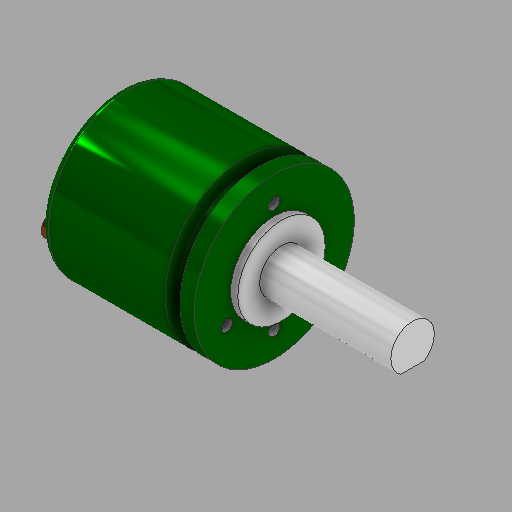
# Autodesk Inventor part: Энкодер P3022-V1-CW360
Saved by Autodesk Inventor 2025 (Build 290162000, 162)
## iProperties
Created: 2025-04-07
Part Number: Энкодер P3022-V1-CW360
Material: Типовые
Document SubType Name: Modeling
Designer: Artem Sannikov
Density: 1 g/cm^3
Appearance: По умолчанию
Author: Artem Sannikov
Autodesk Inventor part; units mm, degrees
ref_plane "YZ Plane" through (0, 0, 0) normal (1, 0, 0) x (0, 1, 0)
ref_plane "XZ Plane" through (0, 0, 0) normal (0, 1, 0) x (-1, 0, 0)
ref_plane "XY Plane" through (0, 0, 0) normal (0, 0, 1) x (1, 0, 0)
sketch "Эскиз1" plane through (0, 0, 0) normal (0, 0, 1) x (1, 0, 0)
  line L0 (0, 0) -> (19.3512, 0) construction
  line L1 (0, 0) -> (0, 11)
  line L2 (0, 11) -> (17, 11)
  line L3 (17, 11) -> (17, 9)
  line L4 (17, 11) -> (17, 9)
  line L5 (17, 9) -> (19, 9)
  line L6 (19, 9) -> (19, 11)
  line L7 (19, 11) -> (21, 11)
  line L8 (21, 11) -> (21, 6)
  line L9 (0, 0) -> (16.5209, 0)
  line L10 (21, 6) -> (22, 6)
  line L11 (22, 6) -> (22, 3)
  line L12 (22, 0) -> (16.5209, 0)
  line L13 (22, 0) -> (40, 0)
  line L14 (40, 0) -> (40, 2.99)
  line L15 (40, 2.99) -> (22, 3)
  dimension "d0" = 11
  dimension "d1" = 2
  dimension "d2" = 2
  dimension "d3" = 2
  dimension "d6" = 5
  dimension "d7" = 1
  dimension "d8" = 17
  dimension "d9" = 18
  dimension "d10" = 2.99
  constraints: 32 end point, 8 perpendicular, 2 collinear, 2 horizontal, 2 vertical, 1 point on line
  measures "d0" distance of L0.start L1.end
  measures "d1" distance of L3.end L2.end
  measures "d2" distance of L3.end L5.end
  measures "d3" distance of L6.end L7.end
  measures "d6" distance between parallel lines of L7 L10
  measures "d7" distance between parallel lines of L8 L11
  measures "d8" distance of L1.end L2.end
  measures "d9" distance of L12.start L13.end
  measures "d10" distance of L13.end L14.end
revolve "Вращение1" add sketch "Эскиз1" angle 360 about axis through (0, 0, 0) along (1, 0, 0)
sketch "Эскиз2" plane through (40, 0, 0) normal (1, 0, 0) x (0, 0, -1)
  line L0 (-1.6248, -2.51) -> (1.6248, -2.51)
  line L1 (-1.6248, -2.51) -> (1.6248, -2.51)
  line L2 (1.6248, -2.51) -> (1.6248, -3.2961)
  line L3 (1.6248, -3.2961) -> (-1.6248, -3.2961)
  line L4 (-1.6248, -3.2961) -> (-1.6248, -2.51)
  point P0 (0, 0)
  point P1 (0, 0)
  constraints: 10 end point, 2 horizontal, 2 parallel, 1 perpendicular
extrude "Выдавливание1" cut sketch "Эскиз2" against normal blind 15
sketch "Эскиз3" plane through (21, 0, 0) normal (1, 0, 0) x (0, 0, -1)
  circle A0 centre (0, 0) radius 7.5 construction
  point P0 (0, 7.5)
  point P1 (-6.4952, -3.75)
  point P2 (6.4952, -3.75)
  point P3 (0, -7.5)
  dimension "d15" = 15
  dimension "d18" = 360
  constraints: 2 point on circle, 1 centre point, 1 coincident, 4 other
  measures "d15" diameter of A0
hole "Отверстие1" at (21, 7.5, 0) at (21, -3.75, 6.4952) at (21, -3.75, -6.4952) at (21, -7.5, 0) direction (-1, 0, 0) diameter 1.567 depth 5 tip angle 118 thread size "M2x0.4" class "6H" standard "ISO Metric profile"
sketch "Эскиз4" plane through (0, 0, 0) normal (-1, 0, 0) x (0, 0, 1)
  line L0 (0, 0) -> (0, -7.5) construction
  circle A0 centre (0, -7.5) radius 1.5
  line L1 (0, 0) -> (6.4952, -3.75) construction
  circle A1 centre (6.4952, -3.75) radius 1.5
  circle A2 centre (-6.4952, -3.75) radius 1.5
  dimension "d27" = 7.5
  dimension "d28" = 3
  dimension "d29" = 7.5
  dimension "d30" = 60
  dimension "d31" = 3
  constraints: 4 end point, 3 centre point, 2 coincident, 1 symmetric about line, 1 vertical, 1 other
  measures "d27" distance of L0.start L0.end
  measures "d28" diameter of A0
  measures "d29" distance of L0.start L1.end
  measures "d30" angle of L0 L1
  measures "d31" diameter of A1
extrude "Выдавливание2" add sketch "Эскиз4" along normal blind 3
fillet "Сопряжение1" radius 1 1 edges at (0, -11, 0)
